Autodesk Fusion 360 part; units mm, degrees
(part 17 of 40)
  spline S18 degree 5 poles (-5.6951, 60.7685) (-5.6979, 60.7993) (-5.7029, 60.8609) (-5.7078, 60.9533) (-5.7097, 61.0766) (-5.7056, 61.231) (-5.6969, 61.3856) (-5.6854, 61.5403) (-5.6723, 61.695) (-5.6583, 61.8498) (-5.6431, 62.0045) (-5.6265, 62.1593) (-5.608, 62.314) (-5.5871, 62.4688) (-5.5641, 62.6235) (-5.539, 62.7782) (-5.5121, 62.9329) (-5.4838, 63.0875) (-5.4542, 63.2421) (-5.4233, 63.3966) (-5.3913, 63.5511) (-5.3579, 63.7055) (-5.3232, 63.8598) (-5.2871, 64.014) (-5.2497, 64.1682) (-5.2109, 64.3222) (-5.1709, 64.4762) (-5.1297, 64.6301) (-5.0873, 64.7839) (-5.0439, 64.9376) (-4.9993, 65.0912) (-4.9536, 65.2447) (-4.9068, 65.398) (-4.8589, 65.5513) (-4.8099, 65.7044) (-4.7599, 65.8574) (-4.7087, 66.0103) (-4.6566, 66.1631) (-4.6035, 66.3158) (-4.5493, 66.4683) (-4.4942, 66.6206) (-4.438, 66.7729) (-4.381, 66.925) (-4.3229, 67.077) (-4.2639, 67.2288) (-4.2039, 67.3804) (-4.143, 67.532) (-4.0812, 67.6833) (-4.0185, 67.8345) (-3.9548, 67.9856) (-3.8903, 68.1365) (-3.8249, 68.2872) (-3.7585, 68.4378) (-3.6913, 68.5882) (-3.6233, 68.7384) (-3.5543, 68.8885) (-3.4846, 69.0384) (-3.4139, 69.1881) (-3.3425, 69.3376) (-3.2701, 69.487) (-3.197, 69.6362) (-3.123, 69.7852) (-3.0482, 69.934) (-2.9726, 70.0826) (-2.8962, 70.2311) (-2.819, 70.3793) (-2.741, 70.5274) (-2.6622, 70.6752) (-2.5826, 70.8229) (-2.5023, 70.9703) (-2.4211, 71.1176) (-2.3556, 71.2352) (-2.3061, 71.3234) (-2.2729, 71.3821) (-2.2563, 71.4115) knots 0 0 0 0 0 0 0.01428571 0.02857143 0.04285714 0.05714286 0.07142857 0.08571429 0.1 0.11428571 0.12857143 0.14285714 0.15714286 0.17142857 0.18571429 0.2 0.21428571 0.22857143 0.24285714 0.25714286 0.27142857 0.28571429 0.3 0.31428571 0.32857143 0.34285714 0.35714286 0.37142857 0.38571429 0.4 0.41428571 0.42857143 0.44285714 0.45714286 0.47142857 0.48571429 0.5 0.51428571 0.52857143 0.54285714 0.55714286 0.57142857 0.58571429 0.6 0.61428571 0.62857143 0.64285714 0.65714286 0.67142857 0.68571429 0.7 0.71428571 0.72857143 0.74285714 0.75714286 0.77142857 0.78571429 0.8 0.81428571 0.82857143 0.84285714 0.85714286 0.87142857 0.88571429 0.9 0.91428571 0.92857143 0.94285714 0.95714286 0.97142857 0.98571429 1 1 1 1 1 1
  arc A47 (2.2563, 71.4115) -> (-2.2563, 71.4115) centre (0, 0) ccw
  spline S19 degree 5 poles (5.6951, 60.7685) (5.6979, 60.7993) (5.7029, 60.8609) (5.7078, 60.9533) (5.7097, 61.0766) (5.7056, 61.231) (5.6969, 61.3856) (5.6854, 61.5403) (5.6723, 61.695) (5.6583, 61.8498) (5.6431, 62.0045) (5.6265, 62.1593) (5.608, 62.314) (5.5871, 62.4688) (5.5641, 62.6235) (5.539, 62.7782) (5.5121, 62.9329) (5.4838, 63.0875) (5.4542, 63.2421) (5.4233, 63.3966) (5.3913, 63.5511) (5.3579, 63.7055) (5.3232, 63.8598) (5.2871, 64.014) (5.2497, 64.1682) (5.2109, 64.3222) (5.1709, 64.4762) (5.1297, 64.6301) (5.0873, 64.7839) (5.0439, 64.9376) (4.9993, 65.0912) (4.9536, 65.2447) (4.9068, 65.398) (4.8589, 65.5513) (4.8099, 65.7044) (4.7599, 65.8574) (4.7087, 66.0103) (4.6566, 66.1631) (4.6035, 66.3158) (4.5493, 66.4683) (4.4942, 66.6206) (4.438, 66.7729) (4.381, 66.925) (4.3229, 67.077) (4.2639, 67.2288) (4.2039, 67.3804) (4.143, 67.532) (4.0812, 67.6833) (4.0185, 67.8345) (3.9548, 67.9856) (3.8903, 68.1365) (3.8249, 68.2872) (3.7585, 68.4378) (3.6913, 68.5882) (3.6233, 68.7384) (3.5543, 68.8885) (3.4846, 69.0384) (3.4139, 69.1881) (3.3425, 69.3376) (3.2701, 69.487) (3.197, 69.6362) (3.123, 69.7852) (3.0482, 69.934) (2.9726, 70.0826) (2.8962, 70.2311) (2.819, 70.3793) (2.741, 70.5274) (2.6622, 70.6752) (2.5826, 70.8229) (2.5023, 70.9703) (2.4211, 71.1176) (2.3556, 71.2352) (2.3061, 71.3234) (2.2729, 71.3821) (2.2563, 71.4115) knots 0 0 0 0 0 0 0.01428571 0.02857143 0.04285714 0.05714286 0.07142857 0.08571429 0.1 0.11428571 0.12857143 0.14285714 0.15714286 0.17142857 0.18571429 0.2 0.21428571 0.22857143 0.24285714 0.25714286 0.27142857 0.28571429 0.3 0.31428571 0.32857143 0.34285714 0.35714286 0.37142857 0.38571429 0.4 0.41428571 0.42857143 0.44285714 0.45714286 0.47142857 0.48571429 0.5 0.51428571 0.52857143 0.54285714 0.55714286 0.57142857 0.58571429 0.6 0.61428571 0.62857143 0.64285714 0.65714286 0.67142857 0.68571429 0.7 0.71428571 0.72857143 0.74285714 0.75714286 0.77142857 0.78571429 0.8 0.81428571 0.82857143 0.84285714 0.85714286 0.87142857 0.88571429 0.9 0.91428571 0.92857143 0.94285714 0.95714286 0.97142857 0.98571429 1 1 1 1 1 1
  spline S20 degree 5 poles (13.3622, 59.5542) (13.369, 59.5843) (13.3833, 59.6444) (13.4071, 59.7338) (13.4435, 59.8517) (13.4951, 59.9973) (13.5511, 60.1416) (13.6099, 60.2852) (13.6701, 60.4283) (13.7313, 60.5711) (13.7935, 60.7136) (13.8571, 60.8557) (13.9226, 60.9971) (13.9902, 61.1379) (14.06, 61.2779) (14.1316, 61.4173) (14.205, 61.5561) (14.2797, 61.6944) (14.3557, 61.8322) (14.4327, 61.9697) (14.5109, 62.1067) (14.5904, 62.2432) (14.6711, 62.3792) (14.753, 62.5148) (14.8363, 62.6498) (14.9208, 62.7843) (15.0064, 62.9184) (15.0932, 63.052) (15.181, 63.1852) (15.2698, 63.318) (15.3597, 63.4503) (15.4506, 63.5821) (15.5425, 63.7135) (15.6354, 63.8445) (15.7293, 63.975) (15.8242, 64.105) (15.92, 64.2346) (16.0168, 64.3638) (16.1146, 64.4926) (16.2132, 64.6209) (16.3127, 64.7488) (16.4131, 64.8762) (16.5144, 65.0032) (16.6166, 65.1298) (16.7196, 65.256) (16.8235, 65.3817) (16.9283, 65.507) (17.0338, 65.6318) (17.1402, 65.7562) (17.2474, 65.8802) (17.3555, 66.0038) (17.4643, 66.1269) (17.5739, 66.2497) (17.6842, 66.3719) (17.7954, 66.4938) (17.9073, 66.6152) (18.02, 66.7362) (18.1335, 66.8568) (18.2477, 66.9769) (18.3626, 67.0966) (18.4782, 67.2159) (18.5946, 67.3347) (18.7118, 67.4531) (18.8296, 67.5711) (18.9481, 67.6887) (19.0674, 67.8058) (19.1873, 67.9225) (19.3079, 68.0388) (19.4293, 68.1546) (19.5512, 68.27) (19.6739, 68.385) (19.7726, 68.4767) (19.8469, 68.5452) (19.8966, 68.5908) (19.9215, 68.6136) knots 0 0 0 0 0 0 0.01428571 0.02857143 0.04285714 0.05714286 0.07142857 0.08571429 0.1 0.11428571 0.12857143 0.14285714 0.15714286 0.17142857 0.18571429 0.2 0.21428571 0.22857143 0.24285714 0.25714286 0.27142857 0.28571429 0.3 0.31428571 0.32857143 0.34285714 0.35714286 0.37142857 0.38571429 0.4 0.41428571 0.42857143 0.44285714 0.45714286 0.47142857 0.48571429 0.5 0.51428571 0.52857143 0.54285714 0.55714286 0.57142857 0.58571429 0.6 0.61428571 0.62857143 0.64285714 0.65714286 0.67142857 0.68571429 0.7 0.71428571 0.72857143 0.74285714 0.75714286 0.77142857 0.78571429 0.8 0.81428571 0.82857143 0.84285714 0.85714286 0.87142857 0.88571429 0.9 0.91428571 0.92857143 0.94285714 0.95714286 0.97142857 0.98571429 1 1 1 1 1 1
  arc A48 (24.2132, 67.2191) -> (19.9215, 68.6136) centre (0, 0) ccw
  spline S21 degree 5 poles (24.1948, 56.0345) (24.2071, 56.0628) (24.2308, 56.1198) (24.264, 56.2062) (24.3039, 56.3229) (24.3478, 56.4711) (24.3873, 56.6208) (24.4241, 56.7714) (24.4595, 56.9226) (24.494, 57.0741) (24.5274, 57.226) (24.5594, 57.3783) (24.5896, 57.5312) (24.6176, 57.6848) (24.6435, 57.8391) (24.6674, 57.994) (24.6897, 58.1494) (24.7105, 58.3052) (24.7301, 58.4614) (24.7485, 58.6179) (24.7658, 58.7747) (24.7818, 58.9318) (24.7965, 59.0893) (24.8098, 59.2471) (24.8218, 59.4053) (24.8325, 59.5638) (24.842, 59.7226) (24.8504, 59.8817) (24.8577, 60.0411) (24.8638, 60.2007) (24.8689, 60.3605) (24.8729, 60.5206) (24.8757, 60.6809) (24.8776, 60.8415) (24.8783, 61.0023) (24.878, 61.1633) (24.8766, 61.3245) (24.8742, 61.4859) (24.8708, 61.6475) (24.8665, 61.8093) (24.8611, 61.9712) (24.8548, 62.1334) (24.8475, 62.2957) (24.8392, 62.4581) (24.83, 62.6207) (24.8199, 62.7835) (24.8088, 62.9464) (24.7967, 63.1095) (24.7838, 63.2727) (24.77, 63.436) (24.7552, 63.5995) (24.7396, 63.7631) (24.723, 63.9268) (24.7056, 64.0906) (24.6873, 64.2545) (24.6681, 64.4185) (24.648, 64.5826) (24.6271, 64.7468) (24.6054, 64.9111) (24.5828, 65.0755) (24.5593, 65.24) (24.535, 65.4046) (24.5098, 65.5692) (24.4839, 65.734) (24.4571, 65.8987) (24.4294, 66.0636) (24.401, 66.2285) (24.3718, 66.3935) (24.3417, 66.5585) (24.3108, 66.7236) (24.2792, 66.8887) (24.2532, 67.0208) (24.2334, 67.1199) (24.22, 67.186) (24.2132, 67.2191) knots 0 0 0 0 0 0 0.01428571 0.02857143 0.04285714 0.05714286 0.07142857 0.08571429 0.1 0.11428571 0.12857143 0.14285714 0.15714286 0.17142857 0.18571429 0.2 0.21428571 0.22857143 0.24285714 0.25714286 0.27142857 0.28571429 0.3 0.31428571 0.32857143 0.34285714 0.35714286 0.37142857 0.38571429 0.4 0.41428571 0.42857143 0.44285714 0.45714286 0.47142857 0.48571429 0.5 0.51428571 0.52857143 0.54285714 0.55714286 0.57142857 0.58571429 0.6 0.61428571 0.62857143 0.64285714 0.65714286 0.67142857 0.68571429 0.7 0.71428571 0.72857143 0.74285714 0.75714286 0.77142857 0.78571429 0.8 0.81428571 0.82857143 0.84285714 0.85714286 0.87142857 0.88571429 0.9 0.91428571 0.92857143 0.94285714 0.95714286 0.97142857 0.98571429 1 1 1 1 1 1
  spline S22 degree 5 poles (31.1115, 52.5103) (31.1272, 52.5368) (31.1594, 52.5895) (31.2097, 52.6672) (31.2807, 52.7681) (31.3748, 52.8906) (31.4727, 53.0106) (31.5729, 53.1289) (31.6744, 53.2464) (31.7767, 53.3634) (31.88, 53.4797) (31.9844, 53.5951) (32.0903, 53.7094) (32.1981, 53.8224) (32.3077, 53.934) (32.419, 54.0444) (32.5316, 54.1537) (32.6455, 54.2622) (32.7603, 54.3698) (32.876, 54.4767) (32.9927, 54.5828) (33.1105, 54.6881) (33.2292, 54.7926) (33.3491, 54.8961) (33.47, 54.9988) (33.5919, 55.1007) (33.7148, 55.2017) (33.8386, 55.302) (33.9633, 55.4015) (34.0888, 55.5003) (34.2151, 55.5984) (34.3423, 55.6957) (34.4703, 55.7923) (34.5991, 55.8881) (34.7288, 55.9832) (34.8592, 56.0776) (34.9905, 56.1712) (35.1224, 56.2642) (35.2552, 56.3564) (35.3886, 56.448) (35.5228, 56.5388) (35.6577, 56.629) (35.7933, 56.7185) (35.9295, 56.8073) (36.0665, 56.8955) (36.2042, 56.9829) (36.3425, 57.0697) (36.4815, 57.1558) (36.6211, 57.2413) (36.7614, 57.3261) (36.9023, 57.4102) (37.0438, 57.4937) (37.186, 57.5765) (37.3288, 57.6587) (37.4721, 57.7403) (37.6161, 57.8212) (37.7607, 57.9014) (37.9058, 57.981) (38.0515, 58.06) (38.1978, 58.1383) (38.3447, 58.216) (38.4921, 58.2931) (38.6401, 58.3695) (38.7886, 58.4453) (38.9377, 58.5205) (39.0873, 58.595) (39.2374, 58.669) (39.3881, 58.7423) (39.5393, 58.8149) (39.6909, 58.887) (39.8431, 58.9584) (39.9653, 59.0151) (40.0572, 59.0573) (40.1185, 59.0853) (40.1492, 59.0993) knots 0 0 0 0 0 0 0.01428571 0.02857143 0.04285714 0.05714286 0.07142857 0.08571429 0.1 0.11428571 0.12857143 0.14285714 0.15714286 0.17142857 0.18571429 0.2 0.21428571 0.22857143 0.24285714 0.25714286 0.27142857 0.28571429 0.3 0.31428571 0.32857143 0.34285714 0.35714286 0.37142857 0.38571429 0.4 0.41428571 0.42857143 0.44285714 0.45714286 0.47142857 0.48571429 0.5 0.51428571 0.52857143 0.54285714 0.55714286 0.57142857 0.58571429 0.6 0.61428571 0.62857143 0.64285714 0.65714286 0.67142857 0.68571429 0.7 0.71428571 0.72857143 0.74285714 0.75714286 0.77142857 0.78571429 0.8 0.81428571 0.82857143 0.84285714 0.85714286 0.87142857 0.88571429 0.9 0.91428571 0.92857143 0.94285714 0.95714286 0.97142857 0.98571429 1 1 1 1 1 1
  arc A49 (43.8, 56.4469) -> (40.1492, 59.0993) centre (0, 0) ccw
  spline S23 degree 5 poles (40.3263, 45.8153) (40.3467, 45.8385) (40.3868, 45.8854) (40.4451, 45.9573) (40.5192, 46.056) (40.6066, 46.1833) (40.6904, 46.3135) (40.772, 46.4454) (40.8524, 46.5782) (40.932, 46.7117) (41.0107, 46.8458) (41.0883, 46.9807) (41.1642, 47.1168) (41.2383, 47.2543) (41.3106, 47.393) (41.3813, 47.5329) (41.4504, 47.6738) (41.5184, 47.8156) (41.5853, 47.9581) (41.6512, 48.1012) (41.716, 48.245) (41.7798, 48.3895) (41.8424, 48.5347) (41.9039, 48.6807) (41.9642, 48.8274) (42.0234, 48.9749) (42.0815, 49.123) (42.1386, 49.2717) (42.1947, 49.421) (42.2499, 49.5709) (42.3041, 49.7214) (42.3574, 49.8724) (42.4097, 50.024) (42.461, 50.1761) (42.5114, 50.3288) (42.5608, 50.482) (42.6094, 50.6358) (42.657, 50.79) (42.7037, 50.9447) (42.7495, 51.0999) (42.7945, 51.2556) (42.8386, 51.4118) (42.8818, 51.5684) (42.9241, 51.7255) (42.9656, 51.883) (43.0063, 52.0409) (43.0461, 52.1993) (43.085, 52.3581) (43.1231, 52.5173) (43.1604, 52.6769) (43.1969, 52.8369) (43.2326, 52.9973) (43.2674, 53.1581) (43.3015, 53.3193) (43.3347, 53.4809) (43.3672, 53.6428) (43.3988, 53.8051) (43.4297, 53.9677) (43.4597, 54.1307) (43.489, 54.294) (43.5175, 54.4577) (43.5453, 54.6217) (43.5723, 54.7861) (43.5984, 54.9508) (43.6239, 55.1158) (43.6486, 55.2811) (43.6725, 55.4467) (43.6956, 55.6126) (43.718, 55.7789) (43.7397, 55.9454) (43.7606, 56.1122) (43.7767, 56.2459) (43.7885, 56.3463) (43.7962, 56.4133) (43.8, 56.4469) knots 0 0 0 0 0 0 0.01428571 0.02857143 0.04285714 0.05714286 0.07142857 0.08571429 0.1 0.11428571 0.12857143 0.14285714 0.15714286 0.17142857 0.18571429 0.2 0.21428571 0.22857143 0.24285714 0.25714286 0.27142857 0.28571429 0.3 0.31428571 0.32857143 0.34285714 0.35714286 0.37142857 0.38571429 0.4 0.41428571 0.42857143 0.44285714 0.45714286 0.47142857 0.48571429 0.5 0.51428571 0.52857143 0.54285714 0.55714286 0.57142857 0.58571429 0.6 0.61428571 0.62857143 0.64285714 0.65714286 0.67142857 0.68571429 0.7 0.71428571 0.72857143 0.74285714 0.75714286 0.77142857 0.78571429 0.8 0.81428571 0.82857143 0.84285714 0.85714286 0.87142857 0.88571429 0.9 0.91428571 0.92857143 0.94285714 0.95714286 0.97142857 0.98571429 1 1 1 1 1 1
  spline S24 degree 5 poles (45.8153, 40.3263) (45.8385, 40.3467) (45.8854, 40.3868) (45.9573, 40.4451) (46.056, 40.5192) (46.1833, 40.6066) (46.3135, 40.6904) (46.4454, 40.772) (46.5782, 40.8524) (46.7117, 40.932) (46.8458, 41.0107) (46.9807, 41.0883) (47.1168, 41.1642) (47.2543, 41.2383) (47.393, 41.3106) (47.5329, 41.3813) (47.6738, 41.4504) (47.8156, 41.5184) (47.9581, 41.5853) (48.1012, 41.6512) (48.245, 41.716) (48.3895, 41.7798) (48.5347, 41.8424) (48.6807, 41.9039) (48.8274, 41.9642) (48.9749, 42.0234) (49.123, 42.0815) (49.2717, 42.1386) (49.421, 42.1947) (49.5709, 42.2499) (49.7214, 42.3041) (49.8724, 42.3574) (50.024, 42.4097) (50.1761, 42.461) (50.3288, 42.5114) (50.482, 42.5608) (50.6358, 42.6094) (50.79, 42.657) (50.9447, 42.7037) (51.0999, 42.7495) (51.2556, 42.7945) (51.4118, 42.8386) (51.5684, 42.8818) (51.7255, 42.9241) (51.883, 42.9656) (52.0409, 43.0063) (52.1993, 43.0461) (52.3581, 43.085) (52.5173, 43.1231) (52.6769, 43.1604) (52.8369, 43.1969) (52.9973, 43.2326) (53.1581, 43.2674) (53.3193, 43.3015) (53.4809, 43.3347) (53.6428, 43.3672) (53.8051, 43.3988) (53.9677, 43.4297) (54.1307, 43.4597) (54.294, 43.489) (54.4577, 43.5175) (54.6217, 43.5453) (54.7861, 43.5723) (54.9508, 43.5984) (55.1158, 43.6239) (55.2811, 43.6486) (55.4467, 43.6725) (55.6126, 43.6956) (55.7789, 43.718) (55.9454, 43.7397) (56.1122, 43.7606) (56.2459, 43.7767) (56.3463, 43.7885) (56.4133, 43.7962) (56.4469, 43.8) knots 0 0 0 0 0 0 0.01428571 0.02857143 0.04285714 0.05714286 0.07142857 0.08571429 0.1 0.11428571 0.12857143 0.14285714 0.15714286 0.17142857 0.18571429 0.2 0.21428571 0.22857143 0.24285714 0.25714286 0.27142857 0.28571429 0.3 0.31428571 0.32857143 0.34285714 0.35714286 0.37142857 0.38571429 0.4 0.41428571 0.42857143 0.44285714 0.45714286 0.47142857 0.48571429 0.5 0.51428571 0.52857143 0.54285714 0.55714286 0.57142857 0.58571429 0.6 0.61428571 0.62857143 0.64285714 0.65714286 0.67142857 0.68571429 0.7 0.71428571 0.72857143 0.74285714 0.75714286 0.77142857 0.78571429 0.8 0.81428571 0.82857143 0.84285714 0.85714286 0.87142857 0.88571429 0.9 0.91428571 0.92857143 0.94285714 0.95714286 0.97142857 0.98571429 1 1 1 1 1 1
  arc A50 (59.0993, 40.1492) -> (56.4469, 43.8) centre (0, 0) ccw
  spline S25 degree 5 poles (52.5103, 31.1115) (52.5368, 31.1272) (52.5895, 31.1594) (52.6672, 31.2097) (52.7681, 31.2807) (52.8906, 31.3748) (53.0106, 31.4727) (53.1289, 31.5729) (53.2464, 31.6744) (53.3634, 31.7767) (53.4797, 31.88) (53.5951, 31.9844) (53.7094, 32.0903) (53.8224, 32.1981) (53.934, 32.3077) (54.0444, 32.419) (54.1537, 32.5316) (54.2622, 32.6455) (54.3698, 32.7603) (54.4767, 32.876) (54.5828, 32.9927) (54.6881, 33.1105) (54.7926, 33.2292) (54.8961, 33.3491) (54.9988, 33.47) (55.1007, 33.5919) (55.2017, 33.7148) (55.302, 33.8386) (55.4015, 33.9633) (55.5003, 34.0888) (55.5984, 34.2151) (55.6957, 34.3423) (55.7923, 34.4703) (55.8881, 34.5991) (55.9832, 34.7288) (56.0776, 34.8592) (56.1712, 34.9905) (56.2642, 35.1224) (56.3564, 35.2552) (56.448, 35.3886) (56.5388, 35.5228) (56.629, 35.6577) (56.7185, 35.7933) (56.8073, 35.9295) (56.8955, 36.0665) (56.9829, 36.2042) (57.0697, 36.3425) (57.1558, 36.4815) (57.2413, 36.6211) (57.3261, 36.7614) (57.4102, 36.9023) (57.4937, 37.0438) (57.5765, 37.186) (57.6587, 37.3288) (57.7403, 37.4721) (57.8212, 37.6161) (57.9014, 37.7607) (57.981, 37.9058) (58.06, 38.0515) (58.1383, 38.1978) (58.216, 38.3447) (58.2931, 38.4921) (58.3695, 38.6401) (58.4453, 38.7886) (58.5205, 38.9377) (58.595, 39.0873) (58.669, 39.2374) (58.7423, 39.3881) (58.8149, 39.5393) (58.887, 39.6909) (58.9584, 39.8431) (59.0151, 39.9653) (59.0573, 40.0572) (59.0853, 40.1185) (59.0993, 40.1492) knots 0 0 0 0 0 0 0.01428571 0.02857143 0.04285714 0.05714286 0.07142857 0.08571429 0.1 0.11428571 0.12857143 0.14285714 0.15714286 0.17142857 0.18571429 0.2 0.21428571 0.22857143 0.24285714 0.25714286 0.27142857 0.28571429 0.3 0.31428571 0.32857143 0.34285714 0.35714286 0.37142857 0.38571429 0.4 0.41428571 0.42857143 0.44285714 0.45714286 0.47142857 0.48571429 0.5 0.51428571 0.52857143 0.54285714 0.55714286 0.57142857 0.58571429 0.6 0.61428571 0.62857143 0.64285714 0.65714286 0.67142857 0.68571429 0.7 0.71428571 0.72857143 0.74285714 0.75714286 0.77142857 0.78571429 0.8 0.81428571 0.82857143 0.84285714 0.85714286 0.87142857 0.88571429 0.9 0.91428571 0.92857143 0.94285714 0.95714286 0.97142857 0.98571429 1 1 1 1 1 1
  spline S26 degree 5 poles (56.0345, 24.1948) (56.0628, 24.2071) (56.1198, 24.2308) (56.2062, 24.264) (56.3229, 24.3039) (56.4711, 24.3478) (56.6208, 24.3873) (56.7714, 24.4241) (56.9226, 24.4595) (57.0741, 24.494) (57.226, 24.5274) (57.3783, 24.5594) (57.5312, 24.5896) (57.6848, 24.6176) (57.8391, 24.6435) (57.994, 24.6674) (58.1494, 24.6897) (58.3052, 24.7105) (58.4614, 24.7301) (58.6179, 24.7485) (58.7747, 24.7658) (58.9318, 24.7818) (59.0893, 24.7965) (59.2471, 24.8098) (59.4053, 24.8218) (59.5638, 24.8325) (59.7226, 24.842) (59.8817, 24.8504) (60.0411, 24.8577) (60.2007, 24.8638) (60.3605, 24.8689) (60.5206, 24.8729) (60.6809, 24.8757) (60.8415, 24.8776) (61.0023, 24.8783) (61.1633, 24.878) (61.3245, 24.8766) (61.4859, 24.8742) (61.6475, 24.8708) (61.8093, 24.8665) (61.9712, 24.8611) (62.1334, 24.8548) (62.2957, 24.8475) (62.4581, 24.8392) (62.6207, 24.83) (62.7835, 24.8199) (62.9464, 24.8088) (63.1095, 24.7967) (63.2727, 24.7838) (63.436, 24.77) (63.5995, 24.7552) (63.7631, 24.7396) (63.9268, 24.723) (64.0906, 24.7056) (64.2545, 24.6873) (64.4185, 24.6681) (64.5826, 24.648) (64.7468, 24.6271) (64.9111, 24.6054) (65.0755, 24.5828) (65.24, 24.5593) (65.4046, 24.535) (65.5692, 24.5098) (65.734, 24.4839) (65.8987, 24.4571) (66.0636, 24.4294) (66.2285, 24.401) (66.3935, 24.3718) (66.5585, 24.3417) (66.7236, 24.3108) (66.8887, 24.2792) (67.0208, 24.2532) (67.1199, 24.2334) (67.186, 24.22) (67.2191, 24.2132) knots 0 0 0 0 0 0 0.01428571 0.02857143 0.04285714 0.05714286 0.07142857 0.08571429 0.1 0.11428571 0.12857143 0.14285714 0.15714286 0.17142857 0.18571429 0.2 0.21428571 0.22857143 0.24285714 0.25714286 0.27142857 0.28571429 0.3 0.31428571 0.32857143 0.34285714 0.35714286 0.37142857 0.38571429 0.4 0.41428571 0.42857143 0.44285714 0.45714286 0.47142857 0.48571429 0.5 0.51428571 0.52857143 0.54285714 0.55714286 0.57142857 0.58571429 0.6 0.61428571 0.62857143 0.64285714 0.65714286 0.67142857 0.68571429 0.7 0.71428571 0.72857143 0.74285714 0.75714286 0.77142857 0.78571429 0.8 0.81428571 0.82857143 0.84285714 0.85714286 0.87142857 0.88571429 0.9 0.91428571 0.92857143 0.94285714 0.95714286 0.97142857 0.98571429 1 1 1 1 1 1
  arc A51 (68.6136, 19.9215) -> (67.2191, 24.2132) centre (0, 0) ccw
  spline S27 degree 5 poles (59.5542, 13.3622) (59.5843, 13.369) (59.6444, 13.3833) (59.7338, 13.4071) (59.8517, 13.4435) (59.9973, 13.4951) (60.1416, 13.5511) (60.2852, 13.6099) (60.4283, 13.6701) (60.5711, 13.7313) (60.7136, 13.7935) (60.8557, 13.8571) (60.9971, 13.9226) (61.1379, 13.9902) (61.2779, 14.06) (61.4173, 14.1316) (61.5561, 14.205) (61.6944, 14.2797) (61.8322, 14.3557) (61.9697, 14.4327) (62.1067, 14.5109) (62.2432, 14.5904) (62.3792, 14.6711) (62.5148, 14.753) (62.6498, 14.8363) (62.7843, 14.9208) (62.9184, 15.0064) (63.052, 15.0932) (63.1852, 15.181) (63.318, 15.2698) (63.4503, 15.3597) (63.5821, 15.4506) (63.7135, 15.5425) (63.8445, 15.6354) (63.975, 15.7293) (64.105, 15.8242) (64.2346, 15.92) (64.3638, 16.0168) (64.4926, 16.1146) (64.6209, 16.2132) (64.7488, 16.3127) (64.8762, 16.4131) (65.0032, 16.5144) (65.1298, 16.6166) (65.256, 16.7196) (65.3817, 16.8235) (65.507, 16.9283) (65.6318, 17.0338) (65.7562, 17.1402) (65.8802, 17.2474) (66.0038, 17.3555) (66.1269, 17.4643) (66.2497, 17.5739) (66.3719, 17.6842) (66.4938, 17.7954) (66.6152, 17.9073) (66.7362, 18.02) (66.8568, 18.1335) (66.9769, 18.2477) (67.0966, 18.3626) (67.2159, 18.4782) (67.3347, 18.5946) (67.4531, 18.7118) (67.5711, 18.8296) (67.6887, 18.9481) (67.8058, 19.0674) (67.9225, 19.1873) (68.0388, 19.3079) (68.1546, 19.4293) (68.27, 19.5512) (68.385, 19.6739) (68.4767, 19.7726) (68.5452, 19.8469) (68.5908, 19.8966) (68.6136, 19.9215) knots 0 0 0 0 0 0 0.01428571 0.02857143 0.04285714 0.05714286 0.07142857 0.08571429 0.1 0.11428571 0.12857143 0.14285714 0.15714286 0.17142857 0.18571429 0.2 0.21428571 0.22857143 0.24285714 0.25714286 0.27142857 0.28571429 0.3 0.31428571 0.32857143 0.34285714 0.35714286 0.37142857 0.38571429 0.4 0.41428571 0.42857143 0.44285714 0.45714286 0.47142857 0.48571429 0.5 0.51428571 0.52857143 0.54285714 0.55714286 0.57142857 0.58571429 0.6 0.61428571 0.62857143 0.64285714 0.65714286 0.67142857 0.68571429 0.7 0.71428571 0.72857143 0.74285714 0.75714286 0.77142857 0.78571429 0.8 0.81428571 0.82857143 0.84285714 0.85714286 0.87142857 0.88571429 0.9 0.91428571 0.92857143 0.94285714 0.95714286 0.97142857 0.98571429 1 1 1 1 1 1
  spline S28 degree 5 poles (60.7685, 5.6951) (60.7993, 5.6979) (60.8609, 5.7029) (60.9533, 5.7078) (61.0766, 5.7097) (61.231, 5.7056) (61.3856, 5.6969) (61.5403, 5.6854) (61.695, 5.6723) (61.8498, 5.6583) (62.0045, 5.6431) (62.1593, 5.6265) (62.314, 5.608) (62.4688, 5.5871) (62.6235, 5.5641) (62.7782, 5.539) (62.9329, 5.5121) (63.0875, 5.4838) (63.2421, 5.4542) (63.3966, 5.4233) (63.5511, 5.3913) (63.7055, 5.3579) (63.8598, 5.3232) (64.014, 5.2871) (64.1682, 5.2497) (64.3222, 5.2109) (64.4762, 5.1709) (64.6301, 5.1297) (64.7839, 5.0873) (64.9376, 5.0439) (65.0912, 4.9993) (65.2447, 4.9536) (65.398, 4.9068) (65.5513, 4.8589) (65.7044, 4.8099) (65.8574, 4.7599) (66.0103, 4.7087) (66.1631, 4.6566) (66.3158, 4.6035) (66.4683, 4.5493) (66.6206, 4.4942) (66.7729, 4.438) (66.925, 4.381) (67.077, 4.3229) (67.2288, 4.2639) (67.3804, 4.2039) (67.532, 4.143) (67.6833, 4.0812) (67.8345, 4.0185) (67.9856, 3.9548) (68.1365, 3.8903) (68.2872, 3.8249) (68.4378, 3.7585) (68.5882, 3.6913) (68.7384, 3.6233) (68.8885, 3.5543) (69.0384, 3.4846) (69.1881, 3.4139) (69.3376, 3.3425) (69.487, 3.2701) (69.6362, 3.197) (69.7852, 3.123) (69.934, 3.0482) (70.0826, 2.9726) (70.2311, 2.8962) (70.3793, 2.819) (70.5274, 2.741) (70.6752, 2.6622) (70.8229, 2.5826) (70.9703, 2.5023) (71.1176, 2.4211) (71.2352, 2.3556) (71.3234, 2.3061) (71.3821, 2.2729) (71.4115, 2.2563) knots 0 0 0 0 0 0 0.01428571 0.02857143 0.04285714 0.05714286 0.07142857 0.08571429 0.1 0.11428571 0.12857143 0.14285714 0.15714286 0.17142857 0.18571429 0.2 0.21428571 0.22857143 0.24285714 0.25714286 0.27142857 0.28571429 0.3 0.31428571 0.32857143 0.34285714 0.35714286 0.37142857 0.38571429 0.4 0.41428571 0.42857143 0.44285714 0.45714286 0.47142857 0.48571429 0.5 0.51428571 0.52857143 0.54285714 0.55714286 0.57142857 0.58571429 0.6 0.61428571 0.62857143 0.64285714 0.65714286 0.67142857 0.68571429 0.7 0.71428571 0.72857143 0.74285714 0.75714286 0.77142857 0.78571429 0.8 0.81428571 0.82857143 0.84285714 0.85714286 0.87142857 0.88571429 0.9 0.91428571 0.92857143 0.94285714 0.95714286 0.97142857 0.98571429 1 1 1 1 1 1
  arc A52 (71.4115, -2.2563) -> (71.4115, 2.2563) centre (0, 0) ccw
  spline S29 degree 5 poles (60.7685, -5.6951) (60.7993, -5.6979) (60.8609, -5.7029) (60.9533, -5.7078) (61.0766, -5.7097) (61.231, -5.7056) (61.3856, -5.6969) (61.5403, -5.6854) (61.695, -5.6723) (61.8498, -5.6583) (62.0045, -5.6431) (62.1593, -5.6265) (62.314, -5.608) (62.4688, -5.5871) (62.6235, -5.5641) (62.7782, -5.539) (62.9329, -5.5121) (63.0875, -5.4838) (63.2421, -5.4542) (63.3966, -5.4233) (63.5511, -5.3913) (63.7055, -5.3579) (63.8598, -5.3232) (64.014, -5.2871) (64.1682, -5.2497) (64.3222, -5.2109) (64.4762, -5.1709) (64.6301, -5.1297) (64.7839, -5.0873) (64.9376, -5.0439) (65.0912, -4.9993) (65.2447, -4.9536) (65.398, -4.9068) (65.5513, -4.8589) (65.7044, -4.8099) (65.8574, -4.7599) (66.0103, -4.7087) (66.1631, -4.6566) (66.3158, -4.6035) (66.4683, -4.5493) (66.6206, -4.4942) (66.7729, -4.438) (66.925, -4.381) (67.077, -4.3229) (67.2288, -4.2639) (67.3804, -4.2039) (67.532, -4.143) (67.6833, -4.0812) (67.8345, -4.0185) (67.9856, -3.9548) (68.1365, -3.8903) (68.2872, -3.8249) (68.4378, -3.7585) (68.5882, -3.6913) (68.7384, -3.6233) (68.8885, -3.5543) (69.0384, -3.4846) (69.1881, -3.4139) (69.3376, -3.3425) (69.487, -3.2701) (69.6362, -3.197) (69.7852, -3.123) (69.934, -3.0482) (70.0826, -2.9726) (70.2311, -2.8962) (70.3793, -2.819) (70.5274, -2.741) (70.6752, -2.6622) (70.8229, -2.5826) (70.9703, -2.5023) (71.1176, -2.4211) (71.2352, -2.3556) (71.3234, -2.3061) (71.3821, -2.2729) (71.4115, -2.2563) knots 0 0 0 0 0 0 0.01428571 0.02857143 0.04285714 0.05714286 0.07142857 0.08571429 0.1 0.11428571 0.12857143 0.14285714 0.15714286 0.17142857 0.18571429 0.2 0.21428571 0.22857143 0.24285714 0.25714286 0.27142857 0.28571429 0.3 0.31428571 0.32857143 0.34285714 0.35714286 0.37142857 0.38571429 0.4 0.41428571 0.42857143 0.44285714 0.45714286 0.47142857 0.48571429 0.5 0.51428571 0.52857143 0.54285714 0.55714286 0.57142857 0.58571429 0.6 0.61428571 0.62857143 0.64285714 0.65714286 0.67142857 0.68571429 0.7 0.71428571 0.72857143 0.74285714 0.75714286 0.77142857 0.78571429 0.8 0.81428571 0.82857143 0.84285714 0.85714286 0.87142857 0.88571429 0.9 0.91428571 0.92857143 0.94285714 0.95714286 0.97142857 0.98571429 1 1 1 1 1 1
  spline S30 degree 5 poles (59.5542, -13.3622) (59.5843, -13.369) (59.6444, -13.3833) (59.7338, -13.4071) (59.8517, -13.4435) (59.9973, -13.4951) (60.1416, -13.5511) (60.2852, -13.6099) (60.4283, -13.6701) (60.5711, -13.7313) (60.7136, -13.7935) (60.8557, -13.8571) (60.9971, -13.9226) (61.1379, -13.9902) (61.2779, -14.06) (61.4173, -14.1316) (61.5561, -14.205) (61.6944, -14.2797) (61.8322, -14.3557) (61.9697, -14.4327) (62.1067, -14.5109) (62.2432, -14.5904) (62.3792, -14.6711) (62.5148, -14.753) (62.6498, -14.8363) (62.7843, -14.9208) (62.9184, -15.0064) (63.052, -15.0932) (63.1852, -15.181) (63.318, -15.2698) (63.4503, -15.3597) (63.5821, -15.4506) (63.7135, -15.5425) (63.8445, -15.6354) (63.975, -15.7293) (64.105, -15.8242) (64.2346, -15.92) (64.3638, -16.0168) (64.4926, -16.1146) (64.6209, -16.2132) (64.7488, -16.3127) (64.8762, -16.4131) (65.0032, -16.5144) (65.1298, -16.6166) (65.256, -16.7196) (65.3817, -16.8235) (65.507, -16.9283) (65.6318, -17.0338) (65.7562, -17.1402) (65.8802, -17.2474) (66.0038, -17.3555) (66.1269, -17.4643) (66.2497, -17.5739) (66.3719, -17.6842) (66.4938, -17.7954) (66.6152, -17.9073) (66.7362, -18.02) (66.8568, -18.1335) (66.9769, -18.2477) (67.0966, -18.3626) (67.2159, -18.4782) (67.3347, -18.5946) (67.4531, -18.7118) (67.5711, -18.8296) (67.6887, -18.9481) (67.8058, -19.0674) (67.9225, -19.1873) (68.0388, -19.3079) (68.1546, -19.4293) (68.27, -19.5512) (68.385, -19.6739) (68.4767, -19.7726) (68.5452, -19.8469) (68.5908, -19.8966) (68.6136, -19.9215) knots 0 0 0 0 0 0 0.01428571 0.02857143 0.04285714 0.05714286 0.07142857 0.08571429 0.1 0.11428571 0.12857143 0.14285714 0.15714286 0.17142857 0.18571429 0.2 0.21428571 0.22857143 0.24285714 0.25714286 0.27142857 0.28571429 0.3 0.31428571 0.32857143 0.34285714 0.35714286 0.37142857 0.38571429 0.4 0.41428571 0.42857143 0.44285714 0.45714286 0.47142857 0.48571429 0.5 0.51428571 0.52857143 0.54285714 0.55714286 0.57142857 0.58571429 0.6 0.61428571 0.62857143 0.64285714 0.65714286 0.67142857 0.68571429 0.7 0.71428571 0.72857143 0.74285714 0.75714286 0.77142857 0.78571429 0.8 0.81428571 0.82857143 0.84285714 0.85714286 0.87142857 0.88571429 0.9 0.91428571 0.92857143 0.94285714 0.95714286 0.97142857 0.98571429 1 1 1 1 1 1
  arc A53 (67.2191, -24.2132) -> (68.6136, -19.9215) centre (0, 0) ccw
  spline S31 degree 5 poles (56.0345, -24.1948) (56.0628, -24.2071) (56.1198, -24.2308) (56.2062, -24.264) (56.3229, -24.3039) (56.4711, -24.3478) (56.6208, -24.3873) (56.7714, -24.4241) (56.9226, -24.4595) (57.0741, -24.494) (57.226, -24.5274) (57.3783, -24.5594) (57.5312, -24.5896) (57.6848, -24.6176) (57.8391, -24.6435) (57.994, -24.6674) (58.1494, -24.6897) (58.3052, -24.7105) (58.4614, -24.7301) (58.6179, -24.7485) (58.7747, -24.7658) (58.9318, -24.7818) (59.0893, -24.7965) (59.2471, -24.8098) (59.4053, -24.8218) (59.5638, -24.8325) (59.7226, -24.842) (59.8817, -24.8504) (60.0411, -24.8577) (60.2007, -24.8638) (60.3605, -24.8689) (60.5206, -24.8729) (60.6809, -24.8757) (60.8415, -24.8776) (61.0023, -24.8783) (61.1633, -24.878) (61.3245, -24.8766) (61.4859, -24.8742) (61.6475, -24.8708) (61.8093, -24.8665) (61.9712, -24.8611) (62.1334, -24.8548) (62.2957, -24.8475) (62.4581, -24.8392) (62.6207, -24.83) (62.7835, -24.8199) (62.9464, -24.8088) (63.1095, -24.7967) (63.2727, -24.7838) (63.436, -24.77) (63.5995, -24.7552) (63.7631, -24.7396) (63.9268, -24.723) (64.0906, -24.7056) (64.2545, -24.6873) (64.4185, -24.6681) (64.5826, -24.648) (64.7468, -24.6271) (64.9111, -24.6054) (65.0755, -24.5828) (65.24, -24.5593) (65.4046, -24.535) (65.5692, -24.5098) (65.734, -24.4839) (65.8987, -24.4571) (66.0636, -24.4294) (66.2285, -24.401) (66.3935, -24.3718) (66.5585, -24.3417) (66.7236, -24.3108) (66.8887, -24.2792) (67.0208, -24.2532) (67.1199, -24.2334) (67.186, -24.22) (67.2191, -24.2132) knots 0 0 0 0 0 0 0.01428571 0.02857143 0.04285714 0.05714286 0.07142857 0.08571429 0.1 0.11428571 0.12857143 0.14285714 0.15714286 0.17142857 0.18571429 0.2 0.21428571 0.22857143 0.24285714 0.25714286 0.27142857 0.28571429 0.3 0.31428571 0.32857143 0.34285714 0.35714286 0.37142857 0.38571429 0.4 0.41428571 0.42857143 0.44285714 0.45714286 0.47142857 0.48571429 0.5 0.51428571 0.52857143 0.54285714 0.55714286 0.57142857 0.58571429 0.6 0.61428571 0.62857143 0.64285714 0.65714286 0.67142857 0.68571429 0.7 0.71428571 0.72857143 0.74285714 0.75714286 0.77142857 0.78571429 0.8 0.81428571 0.82857143 0.84285714 0.85714286 0.87142857 0.88571429 0.9 0.91428571 0.92857143 0.94285714 0.95714286 0.97142857 0.98571429 1 1 1 1 1 1
  spline S32 degree 5 poles (52.5103, -31.1115) (52.5368, -31.1272) (52.5895, -31.1594) (52.6672, -31.2097) (52.7681, -31.2807) (52.8906, -31.3748) (53.0106, -31.4727) (53.1289, -31.5729) (53.2464, -31.6744) (53.3634, -31.7767) (53.4797, -31.88) (53.5951, -31.9844) (53.7094, -32.0903) (53.8224, -32.1981) (53.934, -32.3077) (54.0444, -32.419) (54.1537, -32.5316) (54.2622, -32.6455) (54.3698, -32.7603) (54.4767, -32.876) (54.5828, -32.9927) (54.6881, -33.1105) (54.7926, -33.2292) (54.8961, -33.3491) (54.9988, -33.47) (55.1007, -33.5919) (55.2017, -33.7148) (55.302, -33.8386) (55.4015, -33.9633) (55.5003, -34.0888) (55.5984, -34.2151) (55.6957, -34.3423) (55.7923, -34.4703) (55.8881, -34.5991) (55.9832, -34.7288) (56.0776, -34.8592) (56.1712, -34.9905) (56.2642, -35.1224) (56.3564, -35.2552) (56.448, -35.3886) (56.5388, -35.5228) (56.629, -35.6577) (56.7185, -35.7933) (56.8073, -35.9295) (56.8955, -36.0665) (56.9829, -36.2042) (57.0697, -36.3425) (57.1558, -36.4815) (57.2413, -36.6211) (57.3261, -36.7614) (57.4102, -36.9023) (57.4937, -37.0438) (57.5765, -37.186) (57.6587, -37.3288) (57.7403, -37.4721) (57.8212, -37.6161) (57.9014, -37.7607) (57.981, -37.9058) (58.06, -38.0515) (58.1383, -38.1978) (58.216, -38.3447) (58.2931, -38.4921) (58.3695, -38.6401) (58.4453, -38.7886) (58.5205, -38.9377) (58.595, -39.0873) (58.669, -39.2374) (58.7423, -39.3881) (58.8149, -39.5393) (58.887, -39.6909) (58.9584, -39.8431) (59.0151, -39.9653) (59.0573, -40.0572) (59.0853, -40.1185) (59.0993, -40.1492) knots 0 0 0 0 0 0 0.01428571 0.02857143 0.04285714 0.05714286 0.07142857 0.08571429 0.1 0.11428571 0.12857143 0.14285714 0.15714286 0.17142857 0.18571429 0.2 0.21428571 0.22857143 0.24285714 0.25714286 0.27142857 0.28571429 0.3 0.31428571 0.32857143 0.34285714 0.35714286 0.37142857 0.38571429 0.4 0.41428571 0.42857143 0.44285714 0.45714286 0.47142857 0.48571429 0.5 0.51428571 0.52857143 0.54285714 0.55714286 0.57142857 0.58571429 0.6 0.61428571 0.62857143 0.64285714 0.65714286 0.67142857 0.68571429 0.7 0.71428571 0.72857143 0.74285714 0.75714286 0.77142857 0.78571429 0.8 0.81428571 0.82857143 0.84285714 0.85714286 0.87142857 0.88571429 0.9 0.91428571 0.92857143 0.94285714 0.95714286 0.97142857 0.98571429 1 1 1 1 1 1
  arc A54 (56.4469, -43.8) -> (59.0993, -40.1492) centre (0, 0) ccw
  spline S33 degree 5 poles (45.8153, -40.3263) (45.8385, -40.3467) (45.8854, -40.3868) (45.9573, -40.4451) (46.056, -40.5192) (46.1833, -40.6066) (46.3135, -40.6904) (46.4454, -40.772) (46.5782, -40.8524) (46.7117, -40.932) (46.8458, -41.0107) (46.9807, -41.0883) (47.1168, -41.1642) (47.2543, -41.2383) (47.393, -41.3106) (47.5329, -41.3813) (47.6738, -41.4504) (47.8156, -41.5184) (47.9581, -41.5853) (48.1012, -41.6512) (48.245, -41.716) (48.3895, -41.7798) (48.5347, -41.8424) (48.6807, -41.9039) (48.8274, -41.9642) (48.9749, -42.0234) (49.123, -42.0815) (49.2717, -42.1386) (49.421, -42.1947) (49.5709, -42.2499) (49.7214, -42.3041) (49.8724, -42.3574) (50.024, -42.4097) (50.1761, -42.461) (50.3288, -42.5114) (50.482, -42.5608) (50.6358, -42.6094) (50.79, -42.657) (50.9447, -42.7037) (51.0999, -42.7495) (51.2556, -42.7945) (51.4118, -42.8386) (51.5684, -42.8818) (51.7255, -42.9241) (51.883, -42.9656) (52.0409, -43.0063) (52.1993, -43.0461) (52.3581, -43.085) (52.5173, -43.1231) (52.6769, -43.1604) (52.8369, -43.1969) (52.9973, -43.2326) (53.1581, -43.2674) (53.3193, -43.3015) (53.4809, -43.3347) (53.6428, -43.3672) (53.8051, -43.3988) (53.9677, -43.4297) (54.1307, -43.4597) (54.294, -43.489) (54.4577, -43.5175) (54.6217, -43.5453) (54.7861, -43.5723) (54.9508, -43.5984) (55.1158, -43.6239) (55.2811, -43.6486) (55.4467, -43.6725) (55.6126, -43.6956) (55.7789, -43.718) (55.9454, -43.7397) (56.1122, -43.7606) (56.2459, -43.7767) (56.3463, -43.7885) (56.4133, -43.7962) (56.4469, -43.8) knots 0 0 0 0 0 0 0.01428571 0.02857143 0.04285714 0.05714286 0.07142857 0.08571429 0.1 0.11428571 0.12857143 0.14285714 0.15714286 0.17142857 0.18571429 0.2 0.21428571 0.22857143 0.24285714 0.25714286 0.27142857 0.28571429 0.3 0.31428571 0.32857143 0.34285714 0.35714286 0.37142857 0.38571429 0.4 0.41428571 0.42857143 0.44285714 0.45714286 0.47142857 0.48571429 0.5 0.51428571 0.52857143 0.54285714 0.55714286 0.57142857 0.58571429 0.6 0.61428571 0.62857143 0.64285714 0.65714286 0.67142857 0.68571429 0.7 0.71428571 0.72857143 0.74285714 0.75714286 0.77142857 0.78571429 0.8 0.81428571 0.82857143 0.84285714 0.85714286 0.87142857 0.88571429 0.9 0.91428571 0.92857143 0.94285714 0.95714286 0.97142857 0.98571429 1 1 1 1 1 1
  spline S34 degree 5 poles (40.3263, -45.8153) (40.3467, -45.8385) (40.3868, -45.8854) (40.4451, -45.9573) (40.5192, -46.056) (40.6066, -46.1833) (40.6904, -46.3135) (40.772, -46.4454) (40.8524, -46.5782) (40.932, -46.7117) (41.0107, -46.8458) (41.0883, -46.9807) (41.1642, -47.1168) (41.2383, -47.2543) (41.3106, -47.393) (41.3813, -47.5329) (41.4504, -47.6738) (41.5184, -47.8156) (41.5853, -47.9581) (41.6512, -48.1012) (41.716, -48.245) (41.7798, -48.3895) (41.8424, -48.5347) (41.9039, -48.6807) (41.9642, -48.8274) (42.0234, -48.9749) (42.0815, -49.123) (42.1386, -49.2717) (42.1947, -49.421) (42.2499, -49.5709) (42.3041, -49.7214) (42.3574, -49.8724) (42.4097, -50.024) (42.461, -50.1761) (42.5114, -50.3288) (42.5608, -50.482) (42.6094, -50.6358) (42.657, -50.79) (42.7037, -50.9447) (42.7495, -51.0999) (42.7945, -51.2556) (42.8386, -51.4118) (42.8818, -51.5684) (42.9241, -51.7255) (42.9656, -51.883) (43.0063, -52.0409) (43.0461, -52.1993) (43.085, -52.3581) (43.1231, -52.5173) (43.1604, -52.6769) (43.1969, -52.8369) (43.2326, -52.9973) (43.2674, -53.1581) (43.3015, -53.3193) (43.3347, -53.4809) (43.3672, -53.6428) (43.3988, -53.8051) (43.4297, -53.9677) (43.4597, -54.1307) (43.489, -54.294) (43.5175, -54.4577) (43.5453, -54.6217) (43.5723, -54.7861) (43.5984, -54.9508) (43.6239, -55.1158) (43.6486, -55.2811) (43.6725, -55.4467) (43.6956, -55.6126) (43.718, -55.7789) (43.7397, -55.9454) (43.7606, -56.1122) (43.7767, -56.2459) (43.7885, -56.3463) (43.7962, -56.4133) (43.8, -56.4469) knots 0 0 0 0 0 0 0.01428571 0.02857143 0.04285714 0.05714286 0.07142857 0.08571429 0.1 0.11428571 0.12857143 0.14285714 0.15714286 0.17142857 0.18571429 0.2 0.21428571 0.22857143 0.24285714 0.25714286 0.27142857 0.28571429 0.3 0.31428571 0.32857143 0.34285714 0.35714286 0.37142857 0.38571429 0.4 0.41428571 0.42857143 0.44285714 0.45714286 0.47142857 0.48571429 0.5 0.51428571 0.52857143 0.54285714 0.55714286 0.57142857 0.58571429 0.6 0.61428571 0.62857143 0.64285714 0.65714286 0.67142857 0.68571429 0.7 0.71428571 0.72857143 0.74285714 0.75714286 0.77142857 0.78571429 0.8 0.81428571 0.82857143 0.84285714 0.85714286 0.87142857 0.88571429 0.9 0.91428571 0.92857143 0.94285714 0.95714286 0.97142857 0.98571429 1 1 1 1 1 1
  arc A55 (40.1492, -59.0993) -> (43.8, -56.4469) centre (0, 0) ccw
  spline S35 degree 5 poles (31.1115, -52.5103) (31.1272, -52.5368) (31.1594, -52.5895) (31.2097, -52.6672) (31.2807, -52.7681) (31.3748, -52.8906) (31.4727, -53.0106) (31.5729, -53.1289) (31.6744, -53.2464) (31.7767, -53.3634) (31.88, -53.4797) (31.9844, -53.5951) (32.0903, -53.7094) (32.1981, -53.8224) (32.3077, -53.934) (32.419, -54.0444) (32.5316, -54.1537) (32.6455, -54.2622) (32.7603, -54.3698) (32.876, -54.4767) (32.9927, -54.5828) (33.1105, -54.6881) (33.2292, -54.7926) (33.3491, -54.8961) (33.47, -54.9988) (33.5919, -55.1007) (33.7148, -55.2017) (33.8386, -55.302) (33.9633, -55.4015) (34.0888, -55.5003) (34.2151, -55.5984) (34.3423, -55.6957) (34.4703, -55.7923) (34.5991, -55.8881) (34.7288, -55.9832) (34.8592, -56.0776) (34.9905, -56.1712) (35.1224, -56.2642) (35.2552, -56.3564) (35.3886, -56.448) (35.5228, -56.5388) (35.6577, -56.629) (35.7933, -56.7185) (35.9295, -56.8073) (36.0665, -56.8955) (36.2042, -56.9829) (36.3425, -57.0697) (36.4815, -57.1558) (36.6211, -57.2413) (36.7614, -57.3261) (36.9023, -57.4102) (37.0438, -57.4937) (37.186, -57.5765) (37.3288, -57.6587) (37.4721, -57.7403) (37.6161, -57.8212) (37.7607, -57.9014) (37.9058, -57.981) (38.0515, -58.06) (38.1978, -58.1383) (38.3447, -58.216) (38.4921, -58.2931) (38.6401, -58.3695) (38.7886, -58.4453) (38.9377, -58.5205) (39.0873, -58.595) (39.2374, -58.669) (39.3881, -58.7423) (39.5393, -58.8149) (39.6909, -58.887) (39.8431, -58.9584) (39.9653, -59.0151) (40.0572, -59.0573) (40.1185, -59.0853) (40.1492, -59.0993) knots 0 0 0 0 0 0 0.01428571 0.02857143 0.04285714 0.05714286 0.07142857 0.08571429 0.1 0.11428571 0.12857143 0.14285714 0.15714286 0.17142857 0.18571429 0.2 0.21428571 0.22857143 0.24285714 0.25714286 0.27142857 0.28571429 0.3 0.31428571 0.32857143 0.34285714 0.35714286 0.37142857 0.38571429 0.4 0.41428571 0.42857143 0.44285714 0.45714286 0.47142857 0.48571429 0.5 0.51428571 0.52857143 0.54285714 0.55714286 0.57142857 0.58571429 0.6 0.61428571 0.62857143 0.64285714 0.65714286 0.67142857 0.68571429 0.7 0.71428571 0.72857143 0.74285714 0.75714286 0.77142857 0.78571429 0.8 0.81428571 0.82857143 0.84285714 0.85714286 0.87142857 0.88571429 0.9 0.91428571 0.92857143 0.94285714 0.95714286 0.97142857 0.98571429 1 1 1 1 1 1
  spline S36 degree 5 poles (24.1948, -56.0345) (24.2071, -56.0628) (24.2308, -56.1198) (24.264, -56.2062) (24.3039, -56.3229) (24.3478, -56.4711) (24.3873, -56.6208) (24.4241, -56.7714) (24.4595, -56.9226) (24.494, -57.0741) (24.5274, -57.226) (24.5594, -57.3783) (24.5896, -57.5312) (24.6176, -57.6848) (24.6435, -57.8391) (24.6674, -57.994) (24.6897, -58.1494) (24.7105, -58.3052) (24.7301, -58.4614) (24.7485, -58.6179) (24.7658, -58.7747) (24.7818, -58.9318) (24.7965, -59.0893) (24.8098, -59.2471) (24.8218, -59.4053) (24.8325, -59.5638) (24.842, -59.7226) (24.8504, -59.8817) (24.8577, -60.0411) (24.8638, -60.2007) (24.8689, -60.3605) (24.8729, -60.5206) (24.8757, -60.6809) (24.8776, -60.8415) (24.8783, -61.0023) (24.878, -61.1633) (24.8766, -61.3245) (24.8742, -61.4859) (24.8708, -61.6475) (24.8665, -61.8093) (24.8611, -61.9712) (24.8548, -62.1334) (24.8475, -62.2957) (24.8392, -62.4581) (24.83, -62.6207) (24.8199, -62.7835) (24.8088, -62.9464) (24.7967, -63.1095) (24.7838, -63.2727) (24.77, -63.436) (24.7552, -63.5995) (24.7396, -63.7631) (24.723, -63.9268) (24.7056, -64.0906) (24.6873, -64.2545) (24.6681, -64.4185) (24.648, -64.5826) (24.6271, -64.7468) (24.6054, -64.9111) (24.5828, -65.0755) (24.5593, -65.24) (24.535, -65.4046) (24.5098, -65.5692) (24.4839, -65.734) (24.4571, -65.8987) (24.4294, -66.0636) (24.401, -66.2285) (24.3718, -66.3935) (24.3417, -66.5585) (24.3108, -66.7236) (24.2792, -66.8887) (24.2532, -67.0208) (24.2334, -67.1199) (24.22, -67.186) (24.2132, -67.2191) knots 0 0 0 0 0 0 0.01428571 0.02857143 0.04285714 0.05714286 0.07142857 0.08571429 0.1 0.11428571 0.12857143 0.14285714 0.15714286 0.17142857 0.18571429 0.2 0.21428571 0.22857143 0.24285714 0.25714286 0.27142857 0.28571429 0.3 0.31428571 0.32857143 0.34285714 0.35714286 0.37142857 0.38571429 0.4 0.41428571 0.42857143 0.44285714 0.45714286 0.47142857 0.48571429 0.5 0.51428571 0.52857143 0.54285714 0.55714286 0.57142857 0.58571429 0.6 0.61428571 0.62857143 0.64285714 0.65714286 0.67142857 0.68571429 0.7 0.71428571 0.72857143 0.74285714 0.75714286 0.77142857 0.78571429 0.8 0.81428571 0.82857143 0.84285714 0.85714286 0.87142857 0.88571429 0.9 0.91428571 0.92857143 0.94285714 0.95714286 0.97142857 0.98571429 1 1 1 1 1 1
  arc A56 (19.9215, -68.6136) -> (24.2132, -67.2191) centre (0, 0) ccw
  spline S37 degree 5 poles (13.3622, -59.5542) (13.369, -59.5843) (13.3833, -59.6444) (13.4071, -59.7338) (13.4435, -59.8517) (13.4951, -59.9973) (13.5511, -60.1416) (13.6099, -60.2852) (13.6701, -60.4283) (13.7313, -60.5711) (13.7935, -60.7136) (13.8571, -60.8557) (13.9226, -60.9971) (13.9902, -61.1379) (14.06, -61.2779) (14.1316, -61.4173) (14.205, -61.5561) (14.2797, -61.6944) (14.3557, -61.8322) (14.4327, -61.9697) (14.5109, -62.1067) (14.5904, -62.2432) (14.6711, -62.3792) (14.753, -62.5148) (14.8363, -62.6498) (14.9208, -62.7843) (15.0064, -62.9184) (15.0932, -63.052) (15.181, -63.1852) (15.2698, -63.318) (15.3597, -63.4503) (15.4506, -63.5821) (15.5425, -63.7135) (15.6354, -63.8445) (15.7293, -63.975) (15.8242, -64.105) (15.92, -64.2346) (16.0168, -64.3638) (16.1146, -64.4926) (16.2132, -64.6209) (16.3127, -64.7488) (16.4131, -64.8762) (16.5144, -65.0032) (16.6166, -65.1298) (16.7196, -65.256) (16.8235, -65.3817) (16.9283, -65.507) (17.0338, -65.6318) (17.1402, -65.7562) (17.2474, -65.8802) (17.3555, -66.0038) (17.4643, -66.1269) (17.5739, -66.2497) (17.6842, -66.3719) (17.7954, -66.4938) (17.9073, -66.6152) (18.02, -66.7362) (18.1335, -66.8568) (18.2477, -66.9769) (18.3626, -67.0966) (18.4782, -67.2159) (18.5946, -67.3347) (18.7118, -67.4531) (18.8296, -67.5711) (18.9481, -67.6887) (19.0674, -67.8058) (19.1873, -67.9225) (19.3079, -68.0388) (19.4293, -68.1546) (19.5512, -68.27) (19.6739, -68.385) (19.7726, -68.4767) (19.8469, -68.5452) (19.8966, -68.5908) (19.9215, -68.6136) knots 0 0 0 0 0 0 0.01428571 0.02857143 0.04285714 0.05714286 0.07142857 0.08571429 0.1 0.11428571 0.12857143 0.14285714 0.15714286 0.17142857 0.18571429 0.2 0.21428571 0.22857143 0.24285714 0.25714286 0.27142857 0.28571429 0.3 0.31428571 0.32857143 0.34285714 0.35714286 0.37142857 0.38571429 0.4 0.41428571 0.42857143 0.44285714 0.45714286 0.47142857 0.48571429 0.5 0.51428571 0.52857143 0.54285714 0.55714286 0.57142857 0.58571429 0.6 0.61428571 0.62857143 0.64285714 0.65714286 0.67142857 0.68571429 0.7 0.71428571 0.72857143 0.74285714 0.75714286 0.77142857 0.78571429 0.8 0.81428571 0.82857143 0.84285714 0.85714286 0.87142857 0.88571429 0.9 0.91428571 0.92857143 0.94285714 0.95714286 0.97142857 0.98571429 1 1 1 1 1 1
  circle A57 centre (0, 0) radius 2.3
  arc A58 (-41.8132, -39.3784) -> (-39.3784, -41.8132) centre (0, 0) ccw
  arc A59 (-51.9354, -24.5301) -> (-50.3721, -27.5982) centre (0, 0) ccw
  arc A60 (-56.9737, -7.2806) -> (-56.435, -10.6816) centre (0, 0) ccw
  arc A61 (-56.435, 10.6816) -> (-56.9737, 7.2806) centre (0, 0) ccw
  arc A62 (-50.3721, 27.5982) -> (-51.9354, 24.5301) centre (0, 0) ccw
  arc A63 (-39.3784, 41.8132) -> (-41.8132, 39.3784) centre (0, 0) ccw
  arc A64 (-24.5301, 51.9354) -> (-27.5982, 50.3721) centre (0, 0) ccw
  arc A65 (-7.2806, 56.9737) -> (-10.6816, 56.435) centre (0, 0) ccw
  arc A66 (10.6816, 56.435) -> (7.2806, 56.9737) centre (0, 0) ccw
  arc A67 (27.5982, 50.3721) -> (24.5301, 51.9354) centre (0, 0) ccw
  arc A68 (41.8132, 39.3784) -> (39.3784, 41.8132) centre (0, 0) ccw
  arc A69 (51.9354, 24.5301) -> (50.3721, 27.5982) centre (0, 0) ccw
  arc A70 (56.9737, 7.2806) -> (56.435, 10.6816) centre (0, 0) ccw
  arc A71 (56.435, -10.6816) -> (56.9737, -7.2806) centre (0, 0) ccw
  arc A72 (50.3721, -27.5982) -> (51.9354, -24.5301) centre (0, 0) ccw
  arc A73 (39.3784, -41.8132) -> (41.8132, -39.3784) centre (0, 0) ccw
  arc A74 (24.5301, -51.9354) -> (27.5982, -50.3721) centre (0, 0) ccw
  arc A75 (7.2806, -56.9737) -> (10.6816, -56.435) centre (0, 0) ccw
  arc A76 (7.2806, -56.9737) -> (5.5428, -59.1442) centre (7.5341, -58.9575) ccw
  line L38 (5.5428, -59.1442) -> (5.6951, -60.7685)
  spline S38 degree 5 poles (5.6951, -60.7685) (5.6979, -60.7993) (5.7029, -60.8609) (5.7078, -60.9533) (5.7097, -61.0766) (5.7056, -61.231) (5.6969, -61.3856) (5.6854, -61.5403) (5.6723, -61.695) (5.6583, -61.8498) (5.6431, -62.0045) (5.6265, -62.1593) (5.608, -62.314) (5.5871, -62.4688) (5.5641, -62.6235) (5.539, -62.7782) (5.5121, -62.9329) (5.4838, -63.0875) (5.4542, -63.2421) (5.4233, -63.3966) (5.3913, -63.5511) (5.3579, -63.7055) (5.3232, -63.8598) (5.2871, -64.014) (5.2497, -64.1682) (5.2109, -64.3222) (5.1709, -64.4762) (5.1297, -64.6301) (5.0873, -64.7839) (5.0439, -64.9376) (4.9993, -65.0912) (4.9536, -65.2447) (4.9068, -65.398) (4.8589, -65.5513) (4.8099, -65.7044) (4.7599, -65.8574) (4.7087, -66.0103) (4.6566, -66.1631) (4.6035, -66.3158) (4.5493, -66.4683) (4.4942, -66.6206) (4.438, -66.7729) (4.381, -66.925) (4.3229, -67.077) (4.2639, -67.2288) (4.2039, -67.3804) (4.143, -67.532) (4.0812, -67.6833) (4.0185, -67.8345) (3.9548, -67.9856) (3.8903, -68.1365) (3.8249, -68.2872) (3.7585, -68.4378) (3.6913, -68.5882) (3.6233, -68.7384) (3.5543, -68.8885) (3.4846, -69.0384) (3.4139, -69.1881) (3.3425, -69.3376) (3.2701, -69.487) (3.197, -69.6362) (3.123, -69.7852) (3.0482, -69.934) (2.9726, -70.0826) (2.8962, -70.2311) (2.819, -70.3793) (2.741, -70.5274) (2.6622, -70.6752) (2.5826, -70.8229) (2.5023, -70.9703) (2.4211, -71.1176) (2.3556, -71.2352) (2.3061, -71.3234) (2.2729, -71.3821) (2.2563, -71.4115) knots 0 0 0 0 0 0 0.01428571 0.02857143 0.04285714 0.05714286 0.07142857 0.08571429 0.1 0.11428571 0.12857143 0.14285714 0.15714286 0.17142857 0.18571429 0.2 0.21428571 0.22857143 0.24285714 0.25714286 0.27142857 0.28571429 0.3 0.31428571 0.32857143 0.34285714 0.35714286 0.37142857 0.38571429 0.4 0.41428571 0.42857143 0.44285714 0.45714286 0.47142857 0.48571429 0.5 0.51428571 0.52857143 0.54285714 0.55714286 0.57142857 0.58571429 0.6 0.61428571 0.62857143 0.64285714 0.65714286 0.67142857 0.68571429 0.7 0.71428571 0.72857143 0.74285714 0.75714286 0.77142857 0.78571429 0.8 0.81428571 0.82857143 0.84285714 0.85714286 0.87142857 0.88571429 0.9 0.91428571 0.92857143 0.94285714 0.95714286 0.97142857 0.98571429 1 1 1 1 1 1
  arc A77 (-2.2563, -71.4115) -> (2.2563, -71.4115) centre (0, 0) ccw